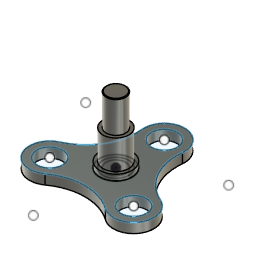
PinGear v0 (Autodesk Fusion 360 design; units mm, degrees)
Autodesk Fusion 360 part; units mm, degrees
sketch "Sketch1" plane through (0, 0, 0) normal (0, 0, 1) x (1, 0, 0)
  circle A0 centre (0, 0) radius 4
  circle A1 centre (0, 0) radius 5
  circle A2 centre (0, 15) radius 4
  circle A3 centre (-12.9904, -7.5) radius 4
  circle A4 centre (12.9904, -7.5) radius 4
  arc A5 (-15.5603, -1.8028) -> (-6.2189, 14.377) centre (-22.1392, 12.7821) ccw
  arc A6 (6.2189, 14.377) -> (15.5603, -1.8028) centre (22.1392, 12.7821) ccw
  arc A7 (6.2189, 14.377) -> (-6.2189, 14.377) centre (0, 15) ccw
  arc A8 (-15.5603, -1.8028) -> (-9.3414, -12.5742) centre (-12.9904, -7.5) ccw
  arc A9 (9.3414, -12.5742) -> (15.5603, -1.8028) centre (12.9904, -7.5) ccw
  arc A10 (9.3414, -12.5742) -> (-9.3414, -12.5742) centre (0, -25.5641) ccw
  circle A11 centre (0, 0) radius 3
  dimension "d1" = 8
  dimension "d2" = 10
  dimension "d3" = 12.5
  dimension "d4" = 15
  dimension "d5" = 8
  dimension "d7" = 360
  dimension "d8" = 32
  dimension "d9" = 32
  dimension "d10" = 32
  dimension "d11" = 6
  constraint coincident A0.centre A1.centre
  constraint concentric A0 A1
  constraint concentric A2 A7
  constraint tangent A6 A7
  constraint tangent A6 A9
  constraint tangent A9 A10
  constraint tangent A8 A10
  constraint tangent A5 A7
  constraint tangent A5 A8
  constraint concentric A0 A11
  measures "d1" diameter of A0
  measures "d2" diameter of A1
  measures "d3" diameter of A7
  measures "d4" distance of A0.centre A2.centre
  measures "d5" diameter of A2
  measures "d8" diameter of A6
  measures "d9" diameter of A10
  measures "d10" diameter of A5
  measures "d11" diameter of A11
extrude "Extrude1" add sketch "Sketch1" along normal blind 20.6 contours A11 makes body 1
extrude "Extrude2" add sketch "Sketch1" along normal blind 10.8 contours A0 bodies 1
extrude "Extrude3" add sketch "Sketch1" along normal blind 1.8 contours A1 bodies 1
extrude "Extrude4" add sketch "Sketch1" against normal blind 3 separate body contours A5 A6 A7 A8 A9 A10 makes body 2
chamfer "Chamfer1" distance 0.2 distance2 0.2 1 edges at (-2.797, -1.0848, 20.6) measured on face at (-1.1591, 0.5829, 20.6) on bodies 1
equation "d12 = 9.8 mm + 9 mm + 1.8 mm"
equation "d14 = 9 mm + 1.8 mm"
